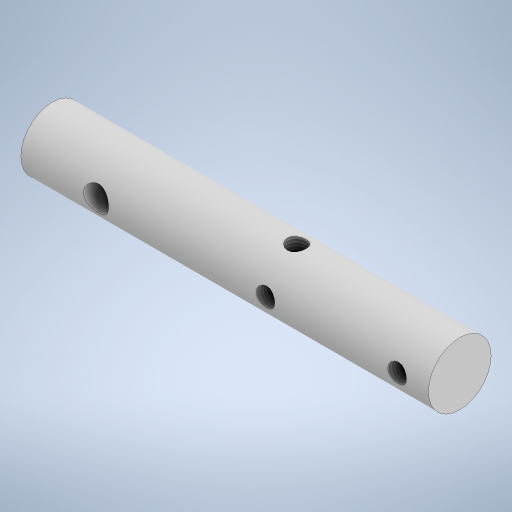
# Autodesk Inventor part: Вал ручки
Saved by Autodesk Inventor 2023 (Build 270158000, 158)
## iProperties
Created: 2022-05-02
Part Number: Вал ручки
Material: Типовые
Document SubType Name: Modeling
Designer: User
Density: 1 g/cm^3
Appearance: По умолчанию
Author: User
Autodesk Inventor part; units mm, degrees
ref_plane "YZ Plane" through (0, 0, 0) normal (1, 0, 0) x (0, 1, 0)
ref_plane "XZ Plane" through (0, 0, 0) normal (0, 1, 0) x (-1, 0, 0)
ref_plane "XY Plane" through (0, 0, 0) normal (0, 0, 1) x (1, 0, 0)
sketch "Эскиз1" plane through (0, 0, 0) normal (1, 0, 0) x (0, 1, 0)
  circle A0 centre (0, 0) radius 5
  dimension "d0" = 10
  constraints: 1 centre point, 1 coincident
  measures "d0" diameter of A0
extrude "Выдавливание1" add sketch "Эскиз1" along normal blind 65
sketch "Эскиз2" plane through (0, 0, 0) normal (0, 0, 1) x (1, 0, 0)
  line L0 (0, 0) -> (12, 0)
  circle A0 centre (12, 0) radius 2
  line L1 (12, 0) -> (29, 0)
  line L2 (29, 0) -> (39, 0)
  circle A1 centre (39, 0) radius 1.5
  dimension "d3" = 12
  dimension "d4" = 4
  dimension "d5" = 17
  dimension "d6" = 10
  dimension "d7" = 3
  constraints: 6 end point, 2 centre point, 2 coincident, 2 horizontal, 1 point on line
  measures "d3" distance of L0.start L0.end
  measures "d4" diameter of A0
  measures "d5" distance of L1.start L1.end
  measures "d6" distance of L1.end L2.end
  measures "d7" diameter of A1
extrude "Выдавливание2" cut sketch "Эскиз2" along normal mid plane 15.25
sketch "Эскиз3" plane through (0, 0, 0) normal (0, 1, 0) x (-1, 0, 0)
  line L0 (-40.5, -5) -> (-40.5, 5) projected
  line L1 (-37.5, -5) -> (-37.5, 5) projected
  line L2 (-37.5, 0) -> (-40.5, 0)
  circle A0 centre (-39, 0) radius 1.5
  point P0 (0, 0)
  dimension "d10" = 3
  constraints: 3 midpoint, 2 end point, 1 centre point
  measures "d10" diameter of A0
extrude "Выдавливание3" cut sketch "Эскиз3" along normal blind 15
thread "Резьба1" size "M3x0.5" class "6H" standard "ISO Metric profile" full length
thread "Резьба2" size "M3x0.5" class "6H" standard "ISO Metric profile" full length
sketch "Эскиз4" plane through (0, 0, 0) normal (0, 0, 1) x (1, 0, 0)
  line L0 (65, -5) -> (65, 5) projected
  line L1 (65, 0) -> (60, 0)
  circle A0 centre (60, 0) radius 1.5
  point P0 (0, 0)
  dimension "d17" = 5
  dimension "d18" = 3
  constraints: 2 end point, 1 centre point, 1 coincident, 1 horizontal, 1 midpoint
  measures "d17" distance of L1.start L1.end
  measures "d18" diameter of A0
extrude "Выдавливание4" cut sketch "Эскиз4" along normal mid plane 21.25
thread "Резьба3" size "M3x0.5" class "6H" standard "ANSI Metric M Profile" full length
sketch "Эскиз5" plane through (0, 0, 0) normal (-1, 0, 0) x (0, 0, 1)
  point P0 (0, 0)
  point P1 (0, 0)
  constraints: 1 coincident
hole "Отверстие1" at (0, 0, 0) direction (1, 0, 0) diameter 2.459 depth 6 tip angle 118 thread size "M3x0.5" class "6H" standard "ISO Metric profile"
